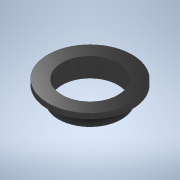
# Autodesk Inventor part: BevelWheelSpace_Clearance
Saved by Autodesk Inventor 2020 (Build 240168000, 168)
## iProperties
Created: 2019-07-10
Part Number: BevelWheelSpace_Clearance
Material: ABS Plastic
Document SubType Name: Modeling
Designer: glesl
Density: 1.06 g/cm^3
Appearance: Glossy - Black
Author: glesl
Autodesk Inventor part; units mm, degrees
ref_plane "YZ Plane" through (0, 0, 0) normal (1, 0, 0) x (0, 1, 0)
ref_plane "XZ Plane" through (0, 0, 0) normal (0, 1, 0) x (-1, 0, 0)
ref_plane "XY Plane" through (0, 0, 0) normal (0, 0, 1) x (1, 0, 0)
sketch "Sketch1" plane through (0, 0, 0) normal (0, 0, 1) x (1, 0, 0)
  line L0 (0, 0) -> (19.05, 0)
  line L1 (19.05, 0) -> (19.05, -2.3622)
  line L2 (19.05, -2.3622) -> (14.8082, -2.3622)
  line L3 (14.8082, -2.3622) -> (14.8082, -8.7122)
  line L4 (14.8082, -8.7122) -> (0, -8.7122)
  line L5 (0, -8.7122) -> (0, 0)
  dimension "d2" = 19.05
  dimension "d3" = 2.3622
  dimension "d4" = 4.2418
  dimension "d5" = 6.35
  constraints: 12 end point, 3 perpendicular, 2 horizontal, 1 vertical
  measures "d2" distance of L0.start L0.end
  measures "d3" distance of L0.end L1.end
  measures "d4" distance of L1.end L2.end
  measures "d5" distance of L2.end L3.end
revolve "Revolution1" add sketch "Sketch1" angle 360 about axis through (0, -8.7122, 0) along (0, 1, 0)
sketch "Sketch2" plane through (0, 0, 0) normal (0, 1, 0) x (1, 0, 0)
  circle A0 centre (0, 0) radius 12.7
  dimension "d7" = 25.4
  constraints: 1 centre point, 1 coincident
  measures "d7" diameter of A0
extrude "Extrusion1" cut sketch "Sketch2" against normal blind 25.4
sketch "Sketch3" plane through (0, -8.7122, 0) normal (0, -1, 0) x (1, 0, 0)
  circle A0 centre (0, 0) radius 14.2875
  circle A1 centre (0, 0) radius 14.8082
  dimension "d10" = 28.575
  constraints: 2 centre point, 2 coincident
  measures "d10" diameter of A0
extrude "Extrusion2" cut sketch "Sketch3" against normal blind 6.35
body "Solid1"
